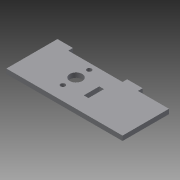
# Autodesk Inventor part: Motor mount plate
Saved by Autodesk Inventor 2015 (Build 190159000, 159)
## iProperties
Created: 2014-07-27
Part Number: Motor mount plate
Material: Generic
Document SubType Name: Modeling
Designer: karl
Density: 1 g/cm^3
Appearance: Default
Author: karl
Autodesk Inventor part; units mm, degrees
ref_plane "YZ Plane" through (0, 0, 0) normal (1, 0, 0) x (0, 1, 0)
ref_plane "XZ Plane" through (0, 0, 0) normal (0, 1, 0) x (-1, 0, 0)
ref_plane "XY Plane" through (0, 0, 0) normal (0, 0, 1) x (1, 0, 0)
sketch "Sketch1" plane through (0, 0, 0) normal (0, 0, 1) x (1, 0, 0)
  circle A0 centre (0, 0) radius 12.5 construction
  circle A1 centre (0, -8.5) radius 1.5 construction
  circle A2 centre (0, 8.5) radius 1.5 construction
  line L0 (-29, -17.5) -> (49, -17.5)
  line L1 (49, -17.5) -> (49, 12.5)
  line L2 (49, 12.5) -> (-29, 12.5)
  line L3 (-29, 12.5) -> (-29, -17.5)
  line L4 (-29, 12.5) -> (-19, 12.5)
  line L5 (-19, 12.5) -> (-19, 15.5)
  line L6 (-19, 15.5) -> (-29, 15.5)
  line L7 (-29, 15.5) -> (-29, 12.5)
  line L8 (10, 12.5) -> (27.5, 12.5)
  line L9 (19, 12.5) -> (29, 12.5)
  line L10 (29, 12.5) -> (29, 15.5)
  line L11 (29, 15.5) -> (19, 15.5)
  line L12 (19, 15.5) -> (19, 12.5)
  line L13 (12.5, 2.5) -> (15.5, 2.5)
  line L14 (15.5, 2.5) -> (15.5, -7.5)
  line L15 (15.5, -7.5) -> (12.5, -7.5)
  line L16 (12.5, -7.5) -> (12.5, 2.5)
  circle A3 centre (0, 0) radius 4
  circle A4 centre (0, -8.5) radius 1.5
  circle A5 centre (0, 8.5) radius 1.5
  point P0 (15.5, -2.5)
  point P1 (49, -2.5)
  dimension "d0" = 25
  dimension "d1" = 3
  dimension "d2" = 3
  dimension "d3" = 17
  dimension "d4" = 8.5
  dimension "d5" = 10
  dimension "d6" = 3
  dimension "d10" = 29
  dimension "d11" = 10
  dimension "d12" = 3
  dimension "d13" = 48
  dimension "d14" = 20
  dimension "d15" = 30
  dimension "d16" = 3
  dimension "d17" = 10
  dimension "d20" = 8
  dimension "d21" = 3
  constraints: 34 end point, 8 parallel, 6 centre point, 5 horizontal, 4 coincident, 4 perpendicular, 3 midpoint, 2 tangent, 2 vertical alignment, 1 concentric, 1 horizontal alignment, 1 point on line
  measures "d0" diameter of A0
  measures "d1" diameter of A1
  measures "d2" diameter of A2
  measures "d3" distance of A2.centre A1.centre
  measures "d4" distance of point (0, 0) A2.centre
  measures "d5" distance of L6.end L5.end
  measures "d6" distance of L5.end L4.end
  measures "d10" distance from line of point (0, 0) L7
  measures "d11" distance of L11.end L10.end
  measures "d12" distance of L10.end L9.end
  measures "d13" distance between parallel lines of L12 L7
  measures "d14" distance between parallel lines of L1 L10
  measures "d15" distance between parallel lines of L2 L0
  measures "d16" distance of L14.end L15.end
  measures "d17" distance of L13.end L14.end
  measures "d20" diameter of A3
  measures "d21" diameter of A4
extrude "Extrusion1" add sketch "Sketch1" along normal blind 3
equation "\"d4\" = 0.5 * d3"
equation "\"d13\" = 2 * d10 - d11"
equation "\"d21\" = d1"
body "Solid1"
